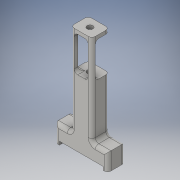
# Autodesk Inventor part: IDISCO-Sampleholder-12mm-60mm
Saved by Autodesk Inventor 2016 (Build 200138000, 138)
## iProperties
Created: 2018-07-25
Part Number: IDISCO-Sampleholder-12mm-60mm
Material: Generic
Document SubType Name: Modeling
Designer: voigt
Density: 1 g/cm^3
Appearance: Default
Author: voigt
Autodesk Inventor part; units mm, degrees
ref_plane "YZ Plane" through (0, 0, 0) normal (1, 0, 0) x (0, 1, 0)
ref_plane "XZ Plane" through (0, 0, 0) normal (0, 1, 0) x (-1, 0, 0)
ref_plane "XY Plane" through (0, 0, 0) normal (0, 0, 1) x (1, 0, 0)
sketch "Sketch1" plane through (0, 0, 0) normal (0, 0, 1) x (1, 0, 0)
  line L0 (0, 7) -> (0, -7) construction
  line L1 (-21, 0) -> (21, 0) construction
  line L2 (-15, 5) -> (15, 5)
  line L3 (15, 5) -> (15, -5)
  line L4 (15, -5) -> (-15, -5)
  line L5 (-15, -5) -> (-15, 5)
  point P0 (0, 0)
  dimension "d0" = 10
  dimension "d1" = 30
  constraints: 8 end point, 2 parallel, 1 horizontal, 1 perpendicular, 2 other
  measures "d0" distance of L2.end L3.end
  measures "d1" distance of L2.start L2.end
extrude "Extrusion1" add sketch "Sketch1" along normal blind 10
sketch "Sketch3" plane through (0, 0, 10) normal (0, 0, 1) x (1, 0, 0)
  line L0 (15, 5) -> (-15, 5) construction
  line L1 (-15, 5) -> (-15, -5) construction
  line L2 (-15, -5) -> (15, -5) construction
  line L3 (15, -5) -> (15, 5) construction
  line L4 (0, 7) -> (0, -7) construction
  line L5 (-21, 0) -> (21, 0) construction
  line L6 (15, 5) -> (-15, 5) projected
  line L7 (-15, -5) -> (15, -5) projected
  line L8 (-6, 5) -> (6, 5)
  line L9 (6, 5) -> (6, -5)
  line L10 (6, -5) -> (-6, -5)
  line L11 (-6, -5) -> (-6, 5)
  point P0 (0, 0)
  dimension "d4" = 12
  constraints: 8 end point, 2 parallel, 2 point on line, 1 horizontal, 1 perpendicular, 1 other
  measures "d4" distance between parallel lines of L9 L11
extrude "Extrusion2" add sketch "Sketch3" along normal blind 52
sketch "Sketch4" plane through (6, -5, 10) normal (1, 0, 0) x (0, 0, -1)
  line L0 (0, 10) -> (0, 0) construction
  line L1 (0, 10) -> (-52, 10) construction
  line L2 (-52, 0) -> (-52, 10) construction
  line L3 (0, 0) -> (-52, 0) construction
  line L4 (0, 10) -> (-52, 10) projected
  line L5 (-50, 10) -> (-30, 10)
  line L6 (-30, 10) -> (-30, 2)
  line L7 (-30, 2) -> (-50, 2)
  line L8 (-50, 2) -> (-50, 10)
  point P0 (10, 5)
  dimension "d7" = 8
  dimension "d8" = 20
  dimension "d9" = 2
  constraints: 8 end point, 2 parallel, 1 horizontal, 1 perpendicular, 1 point on line
  measures "d7" distance between parallel lines of L1 L7
  measures "d8" distance between parallel lines of L8 L6
  measures "d9" distance between parallel lines of L2 L8
extrude "Extrusion3" cut sketch "Sketch4" against normal blind 50
sketch "Sketch5" plane through (0, 0, 0) normal (0, 0, -1) x (-1, 0, 0)
  point P0 (0, 0)
  point P1 (0, 0)
  constraints: 1 coincident
hole "Hole1" at (0, 0, 0) direction (0, 0, 1) diameter 3.3 end through all
sketch "Sketch6" plane through (6, -3, 60) normal (0, 1, 0) x (1, 0, 0)
  line L0 (-12, 0) -> (-12, 20) construction
  line L1 (0, 0) -> (-12, 0) construction
  line L2 (0, 20) -> (0, 0) construction
  line L3 (0, 20) -> (-12, 20) construction
  line L4 (0, 20) -> (-12, 20) projected
  line L5 (-10, 0) -> (-2, 0)
  line L6 (-2, 0) -> (-2, 20)
  line L7 (-2, 20) -> (-10, 20)
  line L8 (-10, 20) -> (-10, 0)
  point P0 (-6, 60)
  dimension "d19" = 2
  dimension "d20" = 2
  constraints: 8 end point, 2 parallel, 2 point on line, 1 horizontal, 1 perpendicular
  measures "d19" distance between parallel lines of L0 L8
  measures "d20" distance between parallel lines of L2 L6
extrude "Extrusion4" cut sketch "Sketch6" against normal up to next
sketch "Sketch7" plane through (-15, 5, 0) normal (0, 1, 0) x (1, 0, 0)
  line L0 (9, -40) -> (21, -40) construction
  line L1 (21, -10) -> (21, -40) construction
  line L2 (30, -10) -> (21, -10) construction
  line L3 (30, 0) -> (30, -10) construction
  line L4 (0, 0) -> (30, 0) construction
  line L5 (0, 0) -> (0, -10) construction
  line L6 (9, -10) -> (0, -10) construction
  line L7 (9, -10) -> (9, -40) construction
  line L8 (30, 0) -> (0, 0) projected
  line L9 (2.5, 0) -> (27.5, 0)
  line L10 (27.5, 0) -> (27.5, -2)
  line L11 (27.5, -2) -> (2.5, -2)
  line L12 (2.5, -2) -> (2.5, 0)
  line L13 (15, 12.4) -> (15, -74.4) construction
  point P0 (15, 0)
  dimension "d23" = 2
  dimension "d24" = 25
  constraints: 8 end point, 2 parallel, 1 horizontal, 1 perpendicular, 1 point on line, 1 other
  measures "d23" distance of L9.end L10.end
  measures "d24" distance between parallel lines of L10 L12
extrude "Extrusion5" cut sketch "Sketch7" against normal up to next
fillet "Fillet1" radius 2 16 edges at (6, 0, 10) (-6, 0, 10) (6, 5, 25) (-6, 5, 25) (-6, -5, 36) (6, -5, 36) (-10.5, 5, 10) (10.5, 5, 10) (10.5, -5, 10) (-10.5, -5, 10) (-15, -5, 5) (-15, 5, 5) (15, 5, 5) (15, -5, 5) (6, 5, 61) (-6, 5, 61)
fillet "Fillet2" radius 2 8 edges at (5, -3, 40) (-5, -3, 40) (-5, -3, 60) (5, -3, 60) (4, -4, 60) (-4, -4, 60) (4, -4, 40) (-4, -4, 40)
body "Solid1"
